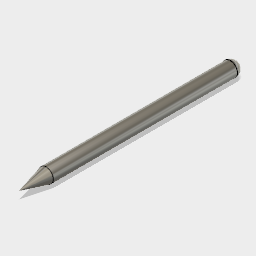
pen v1 (Autodesk Fusion 360 design; units mm, degrees)
Autodesk Fusion 360 part; units mm, degrees
cylinder "圆柱体基本要素1" add diameter 8 height 100 placed x (0, 0, -1) y (0, 1, 0) z (1, 0, 0) at (0, 30, 30) makes body 1
sphere "球体基本要素1" add diameter 8 placed x (0, 0, -1) y (0, 1, 0) z (1, 0, 0) at (0, 20, 43) separate body makes body 2
move_body "对齐1" bodies 1 to x (0, 0, -1) y (0, 1, 0) z (1, 0, 0) at (-30, -10, 143)
sketch "草图4" plane through (0, 0, 0) normal (1, 0, 0) x (0, 0, -1)
sketch "草图5" plane through (0, 0, 0) normal (1, 0, 0) x (0, 0, -1)
  line L0 (0, 1) -> (0, 16)
  line L1 (0, 16) -> (4, 16)
  line L2 (4, 16) -> (0, 1)
revolve "旋转1" add sketch "草图5" angle 360 about axis through (0, 1, 0) along (0, 1, 0) separate body makes body 3
move_body "对齐2" bodies 3 to x (1, 0, 0) y (0, 0, -1) z (0, 1, 0) at (0, 20, 159)
combine "合并1" operation add target body 1 tool bodies 3 2
